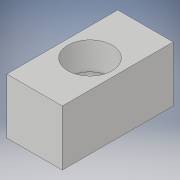
# Autodesk Inventor part: Part3-01
Saved by Autodesk Inventor 2019 (Build 230136000, 136)
## iProperties
Created: 2019-01-18
Part Number: Part3-01
Material: Generic
Document SubType Name: Modeling
Designer: jmc
Density: 1 g/cm^3
Appearance: Default
Author: jmc
Autodesk Inventor part; units mm, degrees
ref_plane "YZ Plane" through (0, 0, 0) normal (1, 0, 0) x (0, 1, 0)
ref_plane "XZ Plane" through (0, 0, 0) normal (0, 1, 0) x (-1, 0, 0)
ref_plane "XY Plane" through (0, 0, 0) normal (0, 0, 1) x (1, 0, 0)
sketch "Sketch1" plane through (0, 0, 0) normal (0, 1, 0) x (-1, 0, 0)
  line L0 (7.9868, 9.2079) -> (-2.0132, 9.2079)
  line L1 (-2.0132, 9.2079) -> (-2.0132, -10.7921)
  line L2 (-2.0132, -10.7921) -> (7.9868, -10.7921)
  line L3 (7.9868, -10.7921) -> (7.9868, 9.2079)
  point P0 (0, 0)
  dimension "height" = 20
  dimension "width" = 10
  constraints: 8 end point, 2 parallel, 1 horizontal, 1 perpendicular
  measures "height" distance of L2.end L0.start
  measures "width" distance of L1.end L2.end
extrude "Extrusion1" add sketch "Sketch1" along normal blind 10
sketch "Sketch2" plane through (0, 10, 0) normal (0, 1, 0) x (1, 0, 0)
  line L0 (-7.9868, 10.7921) -> (-7.9868, -9.2079) construction
  line L1 (-7.9868, 0.7921) -> (2.0132, 0.7921) construction
  line L2 (2.0132, -9.2079) -> (2.0132, 10.7921) construction
  line L3 (-7.9868, -9.2079) -> (2.0132, -9.2079) construction
  line L4 (-2.9868, -9.2079) -> (-2.9868, 10.7921) construction
  line L5 (2.0132, 10.7921) -> (-7.9868, 10.7921) construction
  circle A0 centre (-2.9868, 0.7921) radius 4
  point P0 (0, 0)
  dimension "hole" = 8
  constraints: 5 midpoint, 4 end point, 1 centre point
  measures "hole" diameter of A0
extrude "Extrusion3" cut sketch "Sketch2" against normal blind 5
equation "\"width\" = 0.5 * height"
body "Solid1"
